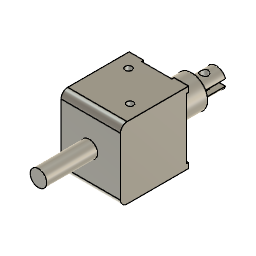
magnet model (Autodesk Fusion 360 design; units mm, degrees)
part number: 2025-10-02-15-07-35-922
part number: 2025-10-02-15-41-49-900
Autodesk Fusion 360 part; units mm, degrees
sketch "Sketch1" plane through (0, 0, 0) normal (1, 0, 0) x (0, 1, 0)
  line L0 (-2.5, 0) -> (-24.15, 0)
  line L1 (-26.65, 2.5) -> (-26.65, 25.45)
  line L2 (-2, 25.45) -> (0, 25.45)
  line L3 (0, 25.45) -> (0, 2.5)
  line L4 (-26.65, 25.45) -> (-24.65, 25.45)
  line L5 (-24.65, 25.45) -> (-24.65, 24.65)
  line L6 (-26.65, 24.65) -> (-26.65, 25.45)
  line L7 (-13.325, 24.65) -> (-13.325, 0) construction
  line L8 (-26.65, 12.725) -> (0, 12.725) construction
  line L9 (-2, 25.45) -> (-2, 24.65)
  line L10 (-24.65, 24.65) -> (-2, 24.65)
  arc A0 (-2.5, 0) -> (0, 2.5) centre (-2.5, 2.5) ccw
  arc A1 (-26.65, 2.5) -> (-24.15, 0) centre (-24.15, 2.5) ccw
  point P0 (-26.65, 0)
  dimension "d1" = 25.45
  dimension "d2" = 26.65
  dimension "d3" = 0.8
  dimension "d4" = 2
  dimension "d5" = 2.5
  constraint horizontal L0
  constraint vertical L1
  constraint horizontal L2
  constraint vertical L3
  constraint horizontal L4
  constraint vertical L5
  constraint vertical L6
  constraint symmetric L4.end L7 L2.start
  constraint symmetric L5.end L7 L9.end
  constraint perpendicular L9 L10
  constraint coincident L10 L7.start
  constraint coincident L0 L7.end
  constraint coincident L3 L8.end
  constraint coincident origin L0
  constraint coincident origin L3
  constraint tangent L0 A0
  constraint tangent L3 A0
  constraint coincident L1 L8.start
  constraint coincident P0 L0
  constraint coincident P0 L1
  constraint tangent L0 A1
  constraint tangent L1 A1
  constraint equal A0 A1
  measures "d1" distance of origin L2.end
  measures "d2" distance of origin P0
  measures "d3" distance of L1.end L6.start
  measures "d4" distance of L5.end L6.start
  measures "d5" radius of A0
extrude "Extrude1" add sketch "Sketch1" along normal blind 22.2 makes body 1
box "BoxPrimitive1" add length 3.835 width 5.425 height 1 placed x (0, 1, 0) y (-1, 0, 0) z (0, 0, 1) at (5.425, -24.65, 24.65) separate body makes body 2
box "BoxPrimitive2" add length 46.471 width 11.3 height 1 placed x (0, -1, 0) y (1, 0, 0) z (0, 0, 1) at (2.9422, -11.5464, 24.65) separate body makes body 3
move_body "Move1" bodies 3 to x (1, 0, 0) y (0, 1, 0) z (0, 0, 1) at (2.4828, 13.9669, 0)
move_body "Move2" bodies 3 to x (1, 0, 0) y (0, 1, 0) z (0, 0, 1) at (0.025, 0, 0)
combine "Combine1" operation cut target body 1 tool bodies 3
copy_body "Body->Comp1" bodies 1 removing the originals makes body 4 in component "Component"
ref_plane "WorkPlane1" through (11.1, -13.325, 12.725) normal (-1, 0, 0) x (0, -1, 0) in component "Component"
ref_plane "WorkPlane1" through (11.1, -13.325, 13.975) normal (0, 1, 0) x (0, 0, 1) in component "Component"
cylinder "CylinderPrimitive1" add diameter 12 height 13 placed x (1, 0, 0) y (0, 1, 0) z (0, 0, 1) at (6.1735, -19.9398, 24.65) separate body makes body 5 in component "Component"
move_body "Move1'" bodies 5 to x (1, 0, 0) y (0, 1, 0) z (0, 0, 1) at (4.9265, 6.6148, 0) in component "Component"
cylinder "CylinderPrimitive2" add diameter 7.4 height 9.2 placed x (1, 0, 0) y (0, 1, 0) z (0, 0, 1) at (11.1, -13.325, 37.65) bodies 5 in component "Component"
box "BoxPrimitive1'" add length 1.2 width 20 height -8 placed x (0, -1, 0) y (1, 0, 0) z (0, 0, 1) at (2.9072, -13.325, 46.85) separate body makes body 6 in component "Component"
mirror "Mirror1" about plane through (11.1, -13.325, 13.975) normal (0, 1, 0) of bodies 6 makes body 7 in component "Component"
combine "Combine1'" operation cut target body 5 tool bodies 6 in component "Component"
combine "Combine2" operation cut target body 5 tool bodies 7 in component "Component"
box "BoxPrimitive2'" add length 6.916 width 7 height -9 placed x (0, 1, 0) y (-1, 0, 0) z (0, 0, 1) at (14.6, -21.4415, 46.85) separate body makes body 8 in component "Component"
hole "Hole1" at (11.1, -21.4415, 42.35) direction (0, 1, 0) diameter 3 depth 25 tip angle 118 bodies 5 8 in component "Component"
combine "Combine3" operation add target body 5 tool bodies 4 in component "Component"
move_body "Move2'" bodies 5 to x (1, 0, 0) y (0, 0, -1) z (0, 1, 0) at (0, -26.65, 8.35) in component "Component"
cylinder "CylinderPrimitive3" add diameter 6.2 height 19 placed x (1, 0, 0) y (0, 0, 1) z (0, -1, 0) at (10.5827, -26.65, 21.675) bodies 5 in component "Component"
cylinder "CylinderPrimitive5" add diameter 2.5 height -2 placed x (1, 0, 0) y (0, 1, 0) z (0, 0, 1) at (22.2, -1.2, 35) separate body makes body 9 in component "Component"
move_body "Move3" bodies 9 to x (1, 0, 0) y (0, 1, 0) z (0, 0, 1) at (-19.45, -3.6, 0) in component "Component"
copy_body "CopyPasteBodies2" bodies 9 makes body 10 in component "Component"
move_body "Move5" bodies 10 to x (1, 0, 0) y (0, 1, 0) z (0, 0, 1) at (19.45, 3.6, 0) in component "Component"
move_body "Move6" bodies 10 to x (1, 0, 0) y (0, 1, 0) z (0, 0, 1) at (-2.75, -16.6, 0) in component "Component"
move_body "Move7" bodies 10 to x (1, 0, 0) y (0, 1, 0) z (0, 0, 1) at (-2.5, 0, 0) in component "Component"
move_body "Move8" bodies 9 to x (1, 0, 0) y (0, 1, 0) z (0, 0, 1) at (2.5, 0, 0) in component "Component"
move_body "Move9" bodies 9 to x (1, 0, 0) y (0, 1, 0) z (0, 0, 1) at (0, -1.865, 0) in component "Component"
combine "Combine5" operation cut target body 5 tool bodies 9 in component "Component"
combine "Combine6" operation cut target body 5 tool bodies 10 in component "Component"
component "Component" placed x (1, 0, 0) y (0, 1, 0) z (0, 0, 1) at (0, 0, 0)
hidden bodies 2 8
